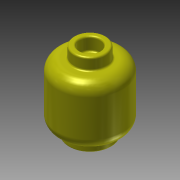
# Autodesk Inventor part: Lego Head
Saved by Autodesk Inventor 2013 (Build 170138000, 138)
## iProperties
Created: 2013-09-06
Part Number: Lego Head
Material: Generic
Document SubType Name: Modeling
Designer: 200395375
Density: 1 g/cm^3
Mass: 0.561108 g
Surface Area: 6.02054 cm^2
Volume: 0.561108 cm^3
Author: 200395375
Autodesk Inventor part; units mm, degrees
ref_plane "YZ Plane" through (0, 0, 0) normal (1, 0, 0) x (0, 1, 0)
ref_plane "XZ Plane" through (0, 0, 0) normal (0, 1, 0) x (-1, 0, 0)
ref_plane "XY Plane" through (0, 0, 0) normal (0, 0, 1) x (1, 0, 0)
sketch "Sketch1" plane through (0, 0, 0) normal (0, 1, 0) x (-1, 0, 0)
  line L0 (0, 0) -> (0, -12.06)
  line L1 (0, 0) -> (2.45, 0)
  line L2 (2.45, 0) -> (2.45, -1.78)
  line L3 (2.45, -1.78) -> (5.01, -1.78)
  line L4 (5.01, -1.78) -> (5.01, -10.85)
  line L5 (5.01, -10.85) -> (3.26, -10.85)
  line L6 (3.26, -10.85) -> (3.26, -12.06)
  line L7 (3.26, -12.06) -> (0, -12.06)
  dimension "d0" = 12.06
  dimension "d1" = 2.45
  dimension "d2" = 1.78
  dimension "d3" = 5.01
  dimension "d4" = 1.21
  dimension "d5" = 3.26
  constraints: 16 end point, 4 perpendicular, 3 parallel, 1 vertical
  measures "d0" distance of L0.start L0.end
  measures "d1" distance of L0.start L1.end
  measures "d2" distance of L1.end L2.end
  measures "d3" distance from line of L0 L3.end
  measures "d4" distance of L5.end L6.end
  measures "d5" distance of L6.end L0.end
revolve "Head" add sketch "Sketch1" angle 360 about axis through (0, 0, 0) along (0, 0, -1)
fillet "Edge" radius 1.75 2 edges at (5.01, 0, -1.78) (5.01, 0, -10.85)
sketch "Sketch2" plane through (0, 0, 0) normal (0, 0, 1) x (1, 0, 0)
  circle A0 centre (0, 0) radius 2.45 projected
  circle A1 centre (0, 0) radius 1.55
  dimension "d8" = 0.9
  constraints: 1 centre point
  measures "d8" radial gap between concentric circles of A0 A1
extrude "Top" cut sketch "Sketch2" against normal blind 2 contours A1
sketch "Sketch3" plane through (0, 0, -12.06) normal (0, 0, -1) x (-1, 0, 0)
  circle A0 centre (0, 0) radius 3.26 projected
  circle A1 centre (0, 0) radius 2.36
  dimension "d11" = 0.9
  constraints: 1 centre point
  measures "d11" radial gap between concentric circles of A1 A0
extrude "Bottom" cut sketch "Sketch3" against normal blind 10 contours A1
fillet "Fillet2" radius 0.25 8 edges at (3.26, 0, -12.06) (3.2601, 0, -10.85) (3.26, 0, -10.85) (2.36, 0, -2.06) (2.45, 0, 0) (-1.55, 0, 0) (-1.55, 0, -2) (2.45, 0, -1.78)
body "Solid1"
